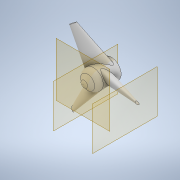
# Autodesk Inventor part: Schiffsschraube
Saved by Autodesk Inventor 2021 (Build 250183000, 183)
## iProperties
Created: 2021-01-08
Part Number: Schiffsschraube
Material: Generisch
Document SubType Name: Modeling
Designer: casa2
Density: 1 g/cm^3
Appearance: Vorgabe
Author: casa2
Autodesk Inventor part; units mm, degrees
ref_plane "XZ Plane" through (0, 0, 0) normal (0, 1, 0) x (-1, 0, 0)
ref_plane "XY Plane" through (0, 0, 0) normal (0, 0, 1) x (1, 0, 0)
sketch "Skizze1" plane through (0, 0, 0) normal (0, 0, 1) x (1, 0, 0)
  circle A0 centre (0, 0) radius 8.5
  circle A1 centre (0, 0) radius 10
  circle A2 centre (0, 0) radius 5
  circle A3 centre (-0.2502, -1.5444) radius 2
  line L0 (-0.0911, 8.4995) -> (0.6371, 8.4761)
  line L1 (8.3262, -1.71) -> (8.1492, -2.4168)
  line L2 (0, 0) -> (-1, 0)
  circle A4 centre (0, 0) radius 6
  line L3 (-6, 0) -> (-5, 0)
  line L4 (-2, -0.8238) -> (-2.1159, -0.8238)
  line L5 (-2, -0.5758) -> (-2, -0.8238)
  line L6 (1.6155, -0.8238) -> (1.9039, -0.8238)
  line L7 (-0.289, 8.4951) -> (-0.289, 8.5059)
  line L8 (-8.5, 0) -> (8.5, 0)
  line L9 (0, 0) -> (0, -8.5)
  line L10 (0, 0) -> (0, 8.4966)
  line L11 (0, 0) -> (0, 1)
  line L12 (0, 1) -> (-8.441, 1)
  line L13 (0, -1) -> (-8.441, -1)
  line L14 (0, 0) -> (-1, 0)
  line L15 (-1, 0) -> (-1, -8.441)
  line L16 (1, 0) -> (1, -8.441)
  line L17 (-1, 0) -> (-1, 8.441)
  line L18 (1, 0) -> (1, 8.441)
  line L19 (0, 1) -> (8.441, 1)
  line L20 (0, -1) -> (8.441, -1)
  point P0 (1.3116, -4.8249)
  point P1 (-0.4922, -4.9757)
  point P2 (-8.4687, 0.7286)
  point P3 (-1.275, 8.4038)
  point P4 (8.4206, 1.1591)
  point P5 (1, -5.9161)
  point P6 (-5.9161, 1)
  point P7 (-1, 5.9161)
  point P8 (-5.9161, -1)
  point P9 (-1, -5.9161)
  point P10 (-8.441, -1)
  point P11 (1, 5.9161)
  point P12 (5.9161, -1)
  point P13 (5.9161, 1)
  dimension "d0" = 17
  dimension "d36" = 12
  dimension "d2" = 10
  dimension "d4" = 4
  dimension "d32" = 20
  dimension "d56" = 1
  dimension "d57" = 1
  constraints: 42 end point, 8 symmetric about line, 6 coincident, 6 point on circle, 3 centre point, 3 horizontal, 3 point on line, 2 perpendicular, 2 vertical, 18 other
  measures "d2" diameter of A2
  measures "d4" diameter of A3
  measures "d32" diameter of A1
  measures "d56" distance of L9.start L11.end
  measures "d57" distance of L9.start L2.end
extrude "Extrusion1" add sketch "Skizze1" along normal blind 22 contours L8 A4 L19 A0 | A0 L20 A4 L8 | L8 A2 L19 A4 | A4 L20 A2 L8 | L18 A4 L10 L0 A0 | L19 A2 L18 A4 | A4 L16 A2 L20 | L18 A2 L10 A4 | L16 A0 L9 A4 | A4 L9 A2 L16 | L0 L10 A4 L17 A0 | L10 A2 L17 A4 | L9 A0 L15 A4 | A4 L15 A2 L9 | L17 A2 L12 A4 | A4 L13 A2 L15 | L12 A2 L3 A4 | A4 L8 A0 L12 | L13 A0 L8 A4 | A4 L3 A2 L13 | A1
ref_plane "Arbeitsebene1" through (0, 0, 29) normal (0, 0, 1) x (1, 0, 0)
sketch "Skizze7" plane through (0, 0, 29) normal (0, 0, 1) x (1, 0, 0)
  circle A0 centre (0, 0) radius 2
  dimension "d38" = 4
  constraints: 1 centre point, 1 coincident
  measures "d38" diameter of A0
loft "Erhebung3" add profiles "Skizze7" section 1 edges at (-10, 0, 22)
fillet "Rundung3" radius 8 1 edges at (-10, 0, 22)
fillet "Rundung4" radius 5 1 edges at (-2, 0, 29)
ref_plane "Arbeitsebene4" through (3.75, 0, 0) normal (1, 0, 0) x (0, 1, 0)
sketch "Skizze8" plane through (3.75, 0, 0) normal (1, 0, 0) x (0, 1, 0)
  line L0 (10, 0) -> (-10, 0) projected
  line L1 (10, 18.3699) -> (-10, 18.3699) projected
  line L2 (0, 0) -> (0, 18.3699)
  ellipse E0 centre (0, 9.1849) end of major axis (-8.6995, 2.453) minor radius 4.9278
  dimension "d46" = 11
  constraints: 2 end point, 2 midpoint, 2 other
ref_plane "Arbeitsebene5" through (43.75, 0, 0) normal (1, 0, 0) x (0, 1, 0)
sketch "Skizze9" plane through (43.75, 0, 0) normal (1, 0, 0) x (0, 1, 0)
  ellipse E0 centre (0, 17.3589) end of major axis (-2.4, 15.5589) minor radius 1.0015
  point P0 (0, 0)
  dimension "d48" = 3
  constraints: 2 other
loft "Erhebung4" add profiles "Skizze8", "Skizze9"
pattern_circular "Runde Anordnung2" count 3 over 360 about axis through (0, 0, 0) along (0, 0, 1) of "Erhebung4"
sketch "Skizze10" plane through (0, 0, 0) normal (0, 0, -1) x (-1, 0, 0)
  circle A0 centre (0, 0) radius 10 projected
  circle A1 centre (0, 0) radius 5 projected
  arc A2 (-8.441, -1) -> (-1, -8.441) centre (0, 0) ccw projected
  arc A3 (1, -8.441) -> (8.441, -1) centre (0, 0) ccw projected
  arc A4 (8.441, 1) -> (1, 8.441) centre (0, 0) ccw projected
  arc A5 (-1, 8.441) -> (-8.441, 1) centre (0, 0) ccw projected
  arc A6 (-5.9161, -1) -> (-1, -5.9161) centre (0, 0) ccw projected
  arc A7 (1, -5.9161) -> (5.9161, -1) centre (0, 0) ccw projected
  line L0 (8.441, -1) -> (5.9161, -1) projected
  line L1 (5.9161, 1) -> (8.441, 1) projected
  arc A8 (5.9161, 1) -> (1, 5.9161) centre (0, 0) ccw projected
  line L2 (1, 8.441) -> (1, 5.9161) projected
  arc A9 (-1, 5.9161) -> (-5.9161, 1) centre (0, 0) ccw projected
  line L3 (-1, 5.9161) -> (-1, 8.441) projected
  line L4 (-8.441, 1) -> (-5.9161, 1) projected
  line L5 (-5.9161, -1) -> (-8.441, -1) projected
  circle A10 centre (0, 0) radius 0.1213 projected
  circle A11 centre (0, 0) radius 5
  line L6 (-8.441, 1) -> (-5.9161, 1)
  line L7 (-0.6371, 8.4761) -> (0.0911, 8.4995) projected
  line L8 (-1, 8.441) -> (-1, 5.9161)
  line L9 (1, 8.441) -> (1, 5.9161) projected
  line L10 (1, 5.9161) -> (1, 8.441)
  arc A12 (8.441, 1) -> (1, 8.441) centre (0, 0) ccw projected
  line L11 (5.9161, 1) -> (8.441, 1) projected
  line L12 (8.441, 1) -> (5.9161, 1)
  line L13 (8.441, -1) -> (5.9161, -1) projected
  line L14 (5.9161, -1) -> (8.441, -1)
  arc A13 (1, -5.9161) -> (5.9161, -1) centre (0, 0) ccw projected
  line L15 (1, -5.9161) -> (1, -8.441)
  line L16 (-5.9161, -1) -> (-8.441, -1)
  line L17 (-1, -5.9161) -> (-1, -8.441)
  arc A14 (-1, 8.441) -> (-8.441, 1) centre (0, 0) ccw
  arc A15 (-1, 5.9161) -> (-5.9161, 1) centre (0, 0) ccw
  arc A16 (5.9161, 1) -> (1, 5.9161) centre (0, 0) ccw projected
  arc A17 (5.9161, 1) -> (1, 5.9161) centre (0, 0) ccw
  arc A18 (8.441, 1) -> (1, 8.441) centre (0, 0) ccw
  arc A19 (1, -8.441) -> (8.441, -1) centre (0, 0) ccw projected
  arc A20 (1, -8.441) -> (8.441, -1) centre (0, 0) ccw
  arc A21 (1, -5.9161) -> (5.9161, -1) centre (0, 0) ccw
  arc A22 (-8.441, -1) -> (-1, -8.441) centre (0, 0) ccw projected
  arc A23 (-8.441, -1) -> (-1, -8.441) centre (0, 0) ccw
  arc A24 (-5.9161, -1) -> (-1, -5.9161) centre (0, 0) ccw projected
  arc A25 (-5.9161, -1) -> (-1, -5.9161) centre (0, 0) ccw
  dimension "d58" = 10
  constraints: 16 end point, 16 point on circle, 9 centre point, 4 concentric, 3 collinear, 2 horizontal, 1 coincident, 1 perpendicular, 1 vertical
  measures "d58" diameter of A11
extrude "Extrusion4" cut sketch "Skizze10" against normal blind 20 contours A1 | L5 A6 L17 A2 | L15 A7 L0 A3 | L1 A8 L2 A4 | L3 A9 L4 A5
equation "\"d0\" = Durchmesser1"
equation "\"d2\" = Durchmesser3"
equation "\"d4\" = Durchmesser4"
equation "\"d32\" = Durchmesser2"
equation "\"d7\" = Größe1"
equation "\"d38\" = Durchmesser5"
equation "\"d43\" = Rundung1"
equation "\"d44\" = Rundung2"
equation "\"d46\" = Ellipse1"
equation "\"d48\" = Ellipse3"
equation "\"Durchmesser1\" = 17"
equation "\"Durchmesser2\" = 20"
equation "\"Durchmesser3\" = 10"
equation "\"Durchmesser4\" = 4"
equation "\"Größe1\" = 22"
equation "\"d9\" = Größe2"
equation "\"Größe2\" = 7"
equation "\"Durchmesser5\" = 4"
equation "\"Rundung2\" = 5"
equation "\"Rundung1\" = 8"
equation "\"Ellipse1\" = 11"
equation "\"Ellipse3\" = 3"
equation "\"d34\" = Durchmesser4"
equation "\"d35\" = Durchmesser4"
